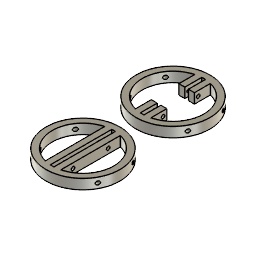
Cactus Needle Booster Avionics Bay Assembly (Autodesk Fusion 360 archive; units mm, degrees)
design "Rocket Mounting Bracket"
part number: 2025-09-21-22-32-14-898
part number: 2025-09-24-11-56-32-151
Autodesk Fusion 360 part; units mm, degrees
sketch "Sketch1" plane through (0, 0, 0) normal (0, 0, 1) x (1, 0, 0)
  circle A0 centre (0, 0) radius 74
  circle A1 centre (0, 0) radius 76
  dimension "d1" = 148
  dimension "d2" = 152
  constraint coincident A0.centre A1.centre
  constraint concentric A0 A1
  measures "d1" diameter of A0
  measures "d2" diameter of A1
extrude "Extrude1" add sketch "Sketch1" along normal blind 300 makes body 1
sketch "Sketch3" plane through (0, 0, 0) normal (0, 0, 1) x (1, 0, 0)
  circle A0 centre (0, 0) radius 73.9
  circle A1 centre (0, 0) radius 61.4
  line L0 (-0.3093, 73.8994) -> (-0.3093, -73.8994)
  line L1 (-0.3093, -73.8994) -> (-0.3093, 73.8994)
  line L2 (-3.9093, 73.8994) -> (-3.9093, -73.8994)
  line L3 (3.2907, -73.8994) -> (3.2907, 73.8994)
  line L4 (3.2907, 73.8994) -> (3.2907, -73.8994)
  line L5 (-3.9093, -73.8994) -> (-3.9093, 73.8994)
  line L6 (-15.9093, 73.8994) -> (-15.9093, -73.8994)
  line L7 (15.2907, 73.8994) -> (15.2907, -73.8994)
  dimension "d5" = 147.8
  dimension "d6" = 122.8
  dimension "d17" = 3.6
  dimension "d18" = -3.6
  dimension "d19" = 12
  dimension "d20" = -12
  constraint coincident A0.centre A1.centre
  constraint coincident A0 L0.start
  constraint coincident A0 L0.end
  constraint vertical L0
  measures "d5" diameter of A0
  measures "d6" diameter of A1
extrude "Extrude2" add sketch "Sketch3" along normal blind 20 separate body contours A0 A1 L7 | A0 A1 L3 L4 L7 | A0 A1 L3 L4 L7 | A0 A1 L0 L1 L3 L4 | A1 L3 L4 L7 | A0 A1 L0 L1 L3 L4 | A0 A1 L0 L1 L2 L5 | A0 A1 L0 L1 L2 L5 | A0 A1 L2 L5 L6 | A0 A1 L2 L5 L6 | A0 A1 L6 | A1 L2 L5 L6 makes body 2
sketch "Sketch5" plane through (-15.9093, 0, 0) normal (-1, 0, 0) x (0, -1, 0)
  line L0 (-59.3031, 0) -> (59.3031, 0)
  line L1 (59.3031, 0) -> (59.3031, 20)
  line L2 (59.3031, 20) -> (-59.3031, 20)
  line L3 (-59.3031, 20) -> (-59.3031, 0)
  line L4 (0, 20) -> (0, 0)
  line L5 (-35.159, 20) -> (-35.159, 0)
  line L6 (35.159, 20) -> (35.159, 0)
  circle A0 centre (-35.159, 10) radius 3.5
  circle A1 centre (35.159, 10) radius 3.5
  dimension "d25" = 35.159
  dimension "d26" = -35.159
  dimension "d27" = 7
  dimension "d28" = 7
  constraint midpoint L2 L4.start
  constraint coincident L4.end origin
  constraint midpoint L5 A0.centre
  constraint midpoint L6 A1.centre
  measures "d27" diameter of A0
  measures "d28" diameter of A1
extrude "Extrude4" cut sketch "Sketch5" against normal blind 190 from surface at 90 contours L5 A0 | L5 A0 | L6 A1 | L6 A1 bodies 2
copy_body "CopyPasteBodies1" bodies 2 makes body 3
move_body "Move1" bodies 3 to x (1, 0, 0) y (0, 1, 0) z (0, 0, 1) at (0, 180, 0)
sketch "Sketch6" plane through (0, 0, 20) normal (0, 0, 1) x (-1, 0, 0)
  arc A0 (-3.2907, -241.3118) -> (3.9093, -241.2754) centre (0, -180) ccw
  line L0 (-3.2907, -241.3118) -> (-3.2907, -118.6882)
  arc A1 (3.9093, -118.7246) -> (-3.2907, -118.6882) centre (0, -180) ccw
  line L1 (3.9093, -118.7246) -> (3.9093, -241.2754)
  arc A2 (15.9093, -239.3031) -> (15.9093, -120.6969) centre (0, -180) ccw
  line L2 (15.9093, -239.3031) -> (15.9093, -120.6969)
  arc A3 (-15.2907, -120.5344) -> (-15.2907, -239.4656) centre (0, -180) ccw
  line L3 (-15.2907, -120.5344) -> (-15.2907, -239.4656)
  circle A4 centre (0, -180) radius 73.9
  line L4 (15.9093, -180) -> (-15.2907, -180)
  line L5 (15.9093, -152.5) -> (-15.2907, -152.5)
  line L6 (15.9093, -207.5) -> (-15.2907, -207.5)
  line L7 (-15.2907, -152.5) -> (-15.2907, -152.9519)
  line L8 (15.9093, -152.5) -> (15.9093, -207.5)
  dimension "d32" = 27.5
  dimension "d33" = -27.5
  constraint midpoint L2 L4.start
  constraint midpoint L3 L4.end
  constraint coincident L3 L7.end
  constraint perpendicular L5 L7
  constraint perpendicular L6 L8
extrude "Extrude5" cut sketch "Sketch6" against normal blind 60 contours L0 L3 L4 L6 | L0 L1 L4 L6 | L1 L2 L4 L6 L8 | L0 L3 L4 L5 L7 | L0 L1 L4 L5 | L1 L2 L4 L5 L8 bodies 3
copy_body "Body->Comp1" bodies 3 removing the originals makes body 4 in component "Component"
component "Component" placed x (1, 0, 0) y (0, 1, 0) z (0, 0, 1) at (0, 0, 0)
hidden bodies 1
equation "d18 = -d17"
equation "d26 = -d25"
equation "d33 = -d32"
